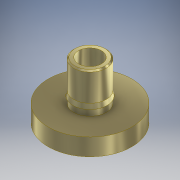
# Autodesk Inventor part: Base
Saved by Autodesk Inventor 2018 (Build 220112000, 112)
## iProperties
Created: 2018-11-03
Part Number: Base
Material: Nickel-Copper Alloy 400
Document SubType Name: Modeling
Designer: Bradley
Density: 8.83 g/cm^3
Appearance: Gold - Metal
Author: Bradley
Autodesk Inventor part; units mm, degrees
ref_plane "YZ Plane" through (0, 0, 0) normal (1, 0, 0) x (0, 1, 0)
ref_plane "XZ Plane" through (0, 0, 0) normal (0, 1, 0) x (-1, 0, 0)
ref_plane "XY Plane" through (0, 0, 0) normal (0, 0, 1) x (1, 0, 0)
sketch "Sketch1" plane through (0, 0, 0) normal (0, 1, 0) x (-1, 0, 0)
  line L0 (0, -0.4064) -> (0, 0.4064)
  line L1 (0, 0.4064) -> (-0.5461, 0.4064)
  line L2 (-0.5461, 0.4064) -> (-0.5461, 2.286)
  line L3 (-0.5461, 2.286) -> (-0.7112, 2.286)
  line L4 (-0.7112, 2.286) -> (-0.7747, 2.2225)
  line L5 (-0.7747, 2.2225) -> (-0.7747, 0.9398)
  line L6 (-0.7747, 0.9398) -> (-0.8128, 0.7112)
  line L7 (-0.8128, 0.7112) -> (-0.7747, 0.7112)
  line L8 (-0.7747, 0.7112) -> (-0.7747, 0.4064)
  line L9 (-0.7747, 0.4064) -> (-1.9812, 0.4064)
  line L10 (-1.9812, 0.4064) -> (-1.9812, -0.4064)
  line L11 (-1.9812, -0.4064) -> (0, -0.4064)
  point P0 (0, 0)
  point P1 (0, 0)
  dimension "d0" = 3.9624
  dimension "d1" = 0.8128
  dimension "d2" = 1.5494
  dimension "d3" = 1.6256
  dimension "d4" = 1.0922
  dimension "d5" = 1.4224
  dimension "d6" = 45
  dimension "d7" = 2.6924
  dimension "d8" = 1.1176
  dimension "d9" = 1.3462
  constraints: 24 end point, 6 perpendicular, 2 point on line, 1 coincident, 1 collinear, 1 horizontal, 1 midpoint, 1 parallel, 1 vertical
  measures "d0" diameter of L10 L0
  measures "d1" distance of L9.end L10.end
  measures "d2" diameter of L8 L0
  measures "d3" diameter of L6.end L0
  measures "d4" diameter of L2 L0
  measures "d5" diameter of L3.end L0
  measures "d6" angle of L4 L3
  measures "d7" distance between parallel lines of L11 L3
  measures "d8" distance between parallel lines of L11 L7
  measures "d9" distance from line of L11 L5.end
revolve "Revolution1" add sketch "Sketch1" angle 360 about axis through (0, 0, -0.4064) along (0, 0, 1)
body "Solid1"
